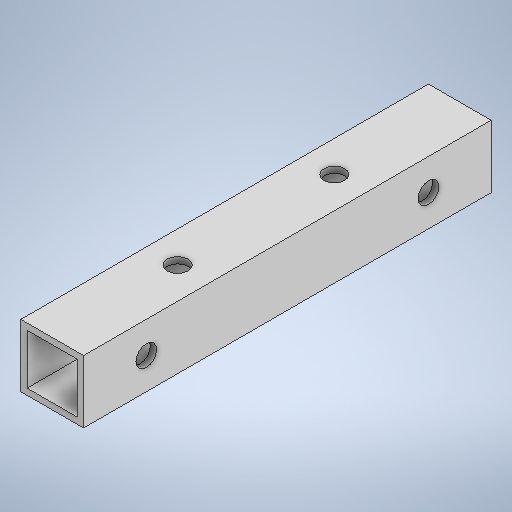
# Autodesk Inventor part: xxkaku_1010
Saved by Autodesk Inventor 2025.1 (Build 291241000, 241)
## iProperties
Created: 2024-12-06
Part Number: xxkaku_1010
Material: 一般
Document SubType Name: Modeling
Designer: yuki0520
Density: 1 g/cm^3
Appearance: 既定
Author: yuki0520
Autodesk Inventor part; units mm, degrees
ref_plane "YZ Plane" through (0, 0, 0) normal (1, 0, 0) x (0, 1, 0)
ref_plane "XZ Plane" through (0, 0, 0) normal (0, 1, 0) x (-1, 0, 0)
ref_plane "XY Plane" through (0, 0, 0) normal (0, 0, 1) x (1, 0, 0)
sketch "スケッチ1" plane through (0, 0, 0) normal (0, 0, 1) x (1, 0, 0)
  line L0 (5, -5) -> (-5, -5)
  line L1 (-5, -5) -> (-5, 5)
  line L2 (-5, 5) -> (5, 5)
  line L3 (5, 5) -> (5, -5)
  line L4 (5, -5) -> (-5, 5) construction
  line L5 (-5, -5) -> (5, 5) construction
  line L6 (4, 4) -> (-4, 4)
  line L7 (-4, 4) -> (-4, -4)
  line L8 (-4, -4) -> (4, -4)
  line L9 (4, -4) -> (4, 4)
  point P0 (0, 0)
  dimension "d0" = 10
  dimension "d1" = 10
  dimension "d2" = 1
  constraints: 20 end point, 4 parallel, 2 midpoint, 2 perpendicular, 1 horizontal, 3 other
  measures "d0" distance of L1.end L2.end
  measures "d1" distance of L2.end L0.start
  measures "d2" distance between parallel lines of L2 L6
extrude "押し出し1" add sketch "スケッチ1" along normal blind 65
sketch "スケッチ2" plane through (5, -5, 0) normal (1, 0, 0) x (0, 0, -1)
  line L0 (0, 5) -> (-65, 5)
  line L1 (-65, 9) -> (-65, 1) projected
  line L2 (0, 0) -> (0, 10) projected
  point P0 (-55, 5)
  point P1 (-10, 5)
  dimension "d5" = 45
  dimension "d6" = 10
  constraints: 2 end point, 2 point on line, 1 midpoint
  measures "d5" distance of point (-55, 5) point (-10, 5)
  measures "d6" distance from line of L2 point (-10, 5)
hole "穴1" at (5, 0, 55) at (5, 0, 10) direction (-1, 0, 0) diameter 3.3 end through all
sketch "スケッチ3" plane through (-5, 5, 0) normal (0, 1, 0) x (1, 0, 0)
  line L0 (5, 0) -> (5, -65)
  line L1 (1, -65) -> (9, -65) projected
  line L2 (10, 0) -> (0, 0) projected
  point P0 (5, -45)
  point P1 (5, -20)
  dimension "d14" = 20
  dimension "d15" = 25
  constraints: 2 end point, 2 point on line, 1 midpoint
  measures "d14" distance from line of L2 point (5, -20)
  measures "d15" distance of point (5, -45) point (5, -20)
hole "穴2" at (0, 5, 45) at (0, 5, 20) direction (0, -1, 0) diameter 3.3 end through all
